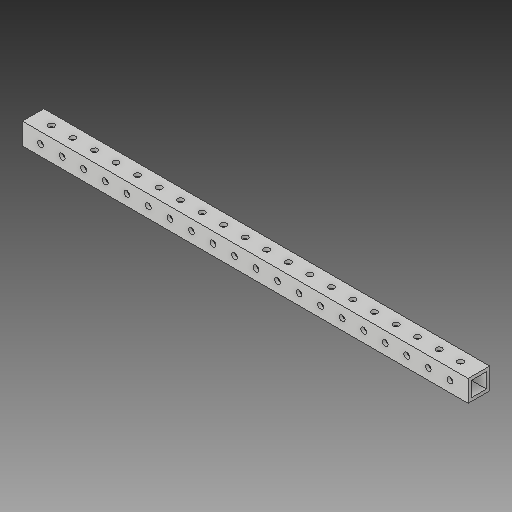
# Autodesk Inventor part: 2020 Extrusion Base
Saved by Autodesk Inventor 2019.4 (Build 234330000, 330)
## iProperties
Created: 2019-12-08
Part Number: 2020 Extrusion Base
Material: Generic
Document SubType Name: Modeling
Designer: admin
Density: 1 g/cm^3
Appearance: Default
Mass: 78.754 g
Surface Area: 570.576 cm^2
Volume: 78.754 cm^3
Author: admin
Autodesk Inventor part; units mm, degrees
ref_plane "YZ Plane" through (0, 0, 0) normal (1, 0, 0) x (0, 1, 0)
ref_plane "XZ Plane" through (0, 0, 0) normal (0, 1, 0) x (-1, 0, 0)
ref_plane "XY Plane" through (0, 0, 0) normal (0, 0, 1) x (1, 0, 0)
sketch "Sketch1" plane through (0, 0, 0) normal (1, 0, 0) x (0, 1, 0)
  line L0 (-10, 10) -> (10, 10)
  line L1 (10, 10) -> (10, -10)
  line L2 (10, -10) -> (-10, -10)
  line L3 (-10, -10) -> (-10, 10)
  line L4 (-10, 10) -> (10, -10) construction
  line L5 (10, 10) -> (-10, -10) construction
  line L6 (7, -7) -> (7, 7)
  line L7 (7, 7) -> (-7, 7)
  line L8 (-7, 7) -> (-7, -7)
  line L9 (-7, -7) -> (7, -7)
  point P0 (0, 0)
  dimension "d0" = 20
  dimension "d1" = 20
  dimension "d2" = 3
  constraints: 20 end point, 4 parallel, 2 midpoint, 2 perpendicular, 1 horizontal, 3 other
  measures "d0" distance of L0.start L0.end
  measures "d1" distance of L0.end L1.end
  measures "d2" distance between parallel lines of L1 L6
extrude "Extrusion1" add sketch "Sketch1" along normal blind 414
sketch "Sketch2" plane through (0, 10, 10) normal (0, 1, 0) x (1, 0, 0)
  circle A0 centre (17, 10) radius 2.75
  line L0 (0, 0) -> (0, 20) projected
  line L1 (0, 0) -> (414, 0) projected
  circle A1 centre (397, 10) radius 2.75
  line L2 (414, 20) -> (414, 0) projected
  circle A2 centre (37, 10) radius 2.75
  circle A3 centre (57, 10) radius 2.75
  circle A4 centre (77, 10) radius 2.75
  circle A5 centre (97, 10) radius 2.75
  circle A6 centre (117, 10) radius 2.75
  circle A7 centre (137, 10) radius 2.75
  circle A8 centre (157, 10) radius 2.75
  circle A9 centre (177, 10) radius 2.75
  circle A10 centre (197, 10) radius 2.75
  circle A11 centre (217, 10) radius 2.75
  circle A12 centre (237, 10) radius 2.75
  circle A13 centre (257, 10) radius 2.75
  circle A14 centre (277, 10) radius 2.75
  circle A15 centre (297, 10) radius 2.75
  circle A16 centre (317, 10) radius 2.75
  circle A17 centre (337, 10) radius 2.75
  circle A18 centre (357, 10) radius 2.75
  circle A19 centre (377, 10) radius 2.75
  circle A20 centre (397, 10) radius 2.75
  point P0 (0, 10)
  dimension "d5" = 5.5
  dimension "d6" = 17
  dimension "d7" = 10
  dimension "d8" = 5.5
  dimension "d9" = 10
  dimension "d10" = 17
  dimension "d13" = 20
  constraints: 21 centre point, 1 horizontal, 38 other
  measures "d5" diameter of A0
  measures "d6" distance from line of L0 A0.centre
  measures "d7" distance from line of L1 A0.centre
  measures "d8" diameter of A1
  measures "d9" distance from line of L1 A1.centre
  measures "d10" distance from line of L2 A1.centre
  measures "d13" distance of A0.centre A2.centre
extrude "Extrusion2" cut sketch "Sketch2" against normal blind 20
sketch "Sketch3" plane through (0, -10, 10) normal (0, 0, 1) x (1, 0, 0)
  circle A0 centre (17, 10) radius 2.75
  line L0 (0, 0) -> (0, 20)
  line L1 (0, 0) -> (414, 0)
  circle A1 centre (397, 10) radius 2.75
  line L2 (414, 20) -> (414, 0)
  circle A2 centre (37, 10) radius 2.75
  circle A3 centre (57, 10) radius 2.75
  circle A4 centre (77, 10) radius 2.75
  circle A5 centre (97, 10) radius 2.75
  circle A6 centre (117, 10) radius 2.75
  circle A7 centre (137, 10) radius 2.75
  circle A8 centre (157, 10) radius 2.75
  circle A9 centre (177, 10) radius 2.75
  circle A10 centre (197, 10) radius 2.75
  circle A11 centre (217, 10) radius 2.75
  circle A12 centre (237, 10) radius 2.75
  circle A13 centre (257, 10) radius 2.75
  circle A14 centre (277, 10) radius 2.75
  circle A15 centre (297, 10) radius 2.75
  circle A16 centre (317, 10) radius 2.75
  circle A17 centre (337, 10) radius 2.75
  circle A18 centre (357, 10) radius 2.75
  circle A19 centre (377, 10) radius 2.75
  circle A20 centre (397, 10) radius 2.75
  point P0 (0, 10)
  dimension "d29" = 5.5
  dimension "d31" = 17
  dimension "d30" = 10
  dimension "d26" = 5.5
  dimension "d28" = 10
  dimension "d27" = 17
  dimension "d21" = 20
  constraints: 21 centre point, 6 end point, 1 horizontal, 38 other
  measures "d29" diameter of A0
  measures "d31" distance from line of L0 A0.centre
  measures "d30" distance from line of L1 A0.centre
  measures "d26" diameter of A1
  measures "d28" distance from line of L1 A1.centre
  measures "d27" distance from line of L2 A1.centre
  measures "d21" distance of A0.centre A2.centre
extrude "Extrusion3" cut sketch "Sketch3" against normal blind 20
body "Solid1"
